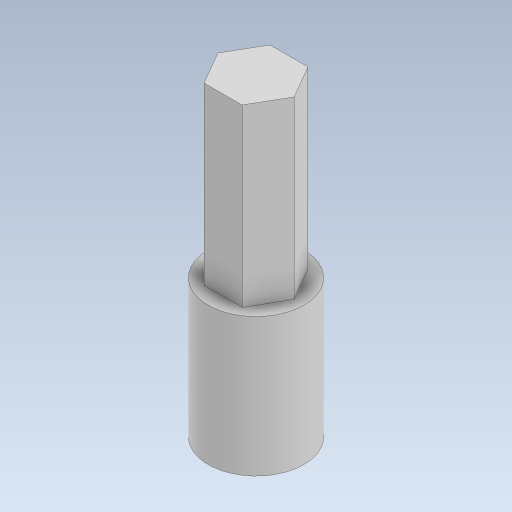
# Autodesk Inventor part: As JGA To Mecanum
Saved by Autodesk Inventor 2023.5 (Build 275446000, 446)
## iProperties
Created: 2025-09-19
Part Number: As JGA To Mecanum
Material: Generic
Document SubType Name: Modeling
Designer: Naufal K
Density: 1 g/cm^3
Appearance: Default
Author: Naufal K
## iProperties of the stored document As JGA To Mecanum 2_3DPrint.ipt
Created: 2025-09-28
Part Number: As JGA To Mecanum 2_3DPrint
Material: Generic
Document SubType Name: Modeling
Designer: Guntur
Density: 1 g/cm^3
Appearance: Default
Author: Guntur
Autodesk Inventor part; units mm, degrees
ref_plane "YZ Plane" through (0, 0, 0) normal (1, 0, 0) x (0, 1, 0)
ref_plane "XZ Plane" through (0, 0, 0) normal (0, 1, 0) x (-1, 0, 0)
ref_plane "XY Plane" through (0, 0, 0) normal (0, 0, 1) x (1, 0, 0)
sketch "Sketch4" plane through (0, 0, 0) normal (0, 1, 0) x (-1, 0, 0)
  circle A0 centre (0, 0) radius 4.5
  dimension "d6" = 9
  constraints: 1 centre point, 1 coincident
  measures "d6" diameter of A0
extrude "Extrusion2" add sketch "Sketch4" along normal blind 13
sketch "Sketch5" plane through (0, 13, 0) normal (0, 1, 0) x (1, 0, 0)
  circle A0 centre (0, 0) radius 2.25
  line L0 (-1.45, -1.7205) -> (-1.45, 1.7205)
  dimension "d9" = 4.5
  dimension "d10" = 3.7
  constraints: 2 end point, 2 point on circle, 1 centre point, 1 coincident, 1 vertical
  measures "d9" diameter of A0
extrude "Extrusion3" cut sketch "Sketch5" against normal blind 13 contours A0 L0 picked at (-0.101, 0.4724)
sketch "Sketch7" plane through (0, 13, 0) normal (0, 1, 0) x (1, 0, 0)
  line L0 (-3.58, 0) -> (-1.79, 3.1004)
  line L1 (-1.79, 3.1004) -> (1.79, 3.1004)
  line L2 (1.79, 3.1004) -> (3.58, 0)
  line L3 (3.58, 0) -> (1.79, -3.1004)
  line L4 (1.79, -3.1004) -> (-1.79, -3.1004)
  line L5 (-1.79, -3.1004) -> (-3.58, 0)
  point P0 (0, 0)
  point P1 (0, 0)
  dimension "d15" = 7.16
  constraints: 12 end point, 1 coincident, 13 other
  measures "d15" distance of L2.end L0.start
extrude "Extrusion5" add sketch "Sketch7" along normal blind 16.5 and the other way blind 0.5
sketch "Sketch15" plane through (-1.45, 0, 1.7205) normal (1, 0, 0) x (0, 0, -1)
  circle A0 centre (1.7748, 6.2834) radius 1
  point P0 (1.7205, 0)
  dimension "d41" = 2
  constraints: 1 centre point
  measures "d41" diameter of A0
extrude "Extrusion11" cut sketch "Sketch15" against normal blind 4.25
sketch "Sketch9" plane through (-1.45, 0, 1.3129) normal (1, 0, 0) x (0, 0, -1)
  circle A0 centre (1.3129, 5.7735) radius 1
  point P0 (1.3129, 0)
  dimension "d21" = 2
  constraints: 1 centre point
  measures "d21" diameter of A0
sketch "Sketch10" plane through (-3.75, 5.7735, 0) normal (-1, 0, 0) x (0, 0, 1)
  point P0 (0, -5.7735)
  point P1 (-0.001, 0.0019)
sketch "Sketch1" plane through (0, 0, 0) normal (0, 1, 0) x (-1, 0, 0)
  circle A0 centre (0, 0) radius 12.5
  dimension "d0" = 25
  dimension "d3" = 4
  dimension "d4" = 7
  dimension "d5" = 3.5
  constraints: 1 centre point, 1 coincident
  measures "d0" diameter of A0
body "Solid1"
body "Solid2"
